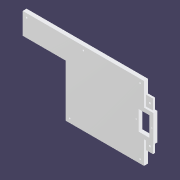
# Autodesk Inventor part: SP001b
Saved by Autodesk Inventor 2017 SP1 (Build 210196100, 196)
## iProperties
Created: 2018-01-11
Part Number: SP001b
Material: ABS Plastic
Document SubType Name: Modeling
Designer: Zach
Density: 1.06 g/cm^3
Appearance: CR White
Mass: 551.84 g
Surface Area: 1185.09 cm^2
Volume: 520.604 cm^3
Author: Zach
Autodesk Inventor part; units mm, degrees
ref_plane "YZ Plane" through (0, 0, 0) normal (1, 0, 0) x (0, 1, 0)
ref_plane "XZ Plane" through (0, 0, 0) normal (0, 1, 0) x (-1, 0, 0)
ref_plane "XY Plane" through (0, 0, 0) normal (0, 0, 1) x (1, 0, 0)
sketch "Sketch1" plane through (0, 0, 0) normal (0, 0, 1) x (1, 0, 0)
  line L0 (0, 0) -> (620, 0)
  line L1 (110, -188) -> (510, -188)
  line L2 (510, -188) -> (510, -55)
  line L3 (510, -55) -> (620, -55)
  line L4 (620, -55) -> (620, 0)
  line L5 (110, -188) -> (110, -55)
  line L6 (0, -55) -> (0, 0)
  line L7 (0, -55) -> (110, -55)
  point P0 (310, -188)
  point P1 (310, 0)
  dimension "d0" = 620
  dimension "d1" = 188
  dimension "d2" = 400
  dimension "d3" = 133
  constraints: 16 end point, 3 perpendicular, 2 horizontal, 2 midpoint, 2 parallel, 2 point on line, 1 vertical, 1 vertical alignment
  measures "d0" distance of L0.start L0.end
  measures "d1" distance between parallel lines of L0 L1
  measures "d2" distance of L1.start L1.end
  measures "d3" distance of L1.end L2.end
extrude "Extrusion1" add sketch "Sketch1" along normal blind 10
sketch "Sketch2" plane through (0, 0, 10) normal (0, 0, 1) x (1, 0, 0)
  line L0 (620, 0) -> (0, 0) projected
  line L1 (510, -188) -> (110, -188) projected
  line L2 (620, 0) -> (310, 0)
  line L3 (310, 0) -> (310, -188)
  line L4 (310, -188) -> (620, -188)
  line L5 (620, -188) -> (620, 0)
  constraints: 8 end point, 2 parallel, 1 horizontal, 1 midpoint, 1 perpendicular
extrude "Extrusion2" cut sketch "Sketch2" against normal through all
sketch "Sketch3" plane through (0, 0, 10) normal (0, 0, 1) x (1, 0, 0)
  circle A0 centre (10, -10) radius 2
  line L0 (310, 0) -> (0, 0) projected
  line L1 (0, 0) -> (0, -55) projected
  circle A1 centre (155, -10) radius 2
  circle A2 centre (300, -10) radius 2
  line L2 (310, -188) -> (310, 0) projected
  line L3 (10, -10) -> (300, -10) construction
  circle A3 centre (120, -178) radius 2
  line L4 (110, -55) -> (110, -188) projected
  line L5 (110, -188) -> (310, -188) projected
  circle A4 centre (300, -178) radius 2
  dimension "d8" = 4
  dimension "d9" = 10
  dimension "d10" = 10
  dimension "d11" = 4
  dimension "d12" = 4
  dimension "d13" = 10
  dimension "d14" = 4
  dimension "d15" = 10
  dimension "d16" = 10
  dimension "d17" = 4
  dimension "d18" = 10
  dimension "d19" = 10
  constraints: 5 centre point, 2 end point, 2 horizontal alignment, 1 coincident, 1 horizontal, 1 midpoint
  measures "d8" diameter of A0
  measures "d9" distance from line of L0 L3.start
  measures "d10" distance from line of L1 L3.start
  measures "d11" diameter of A1
  measures "d12" diameter of A2
  measures "d13" distance from line of L2 L3.end
  measures "d14" diameter of A3
  measures "d15" distance from line of L4 A3.centre
  measures "d16" distance from line of L5 A3.centre
  measures "d17" diameter of A4
  measures "d18" distance from line of L2 A4.centre
  measures "d19" distance from line of L5 A4.centre
extrude "Extrusion3" cut sketch "Sketch3" against normal through all
sketch "Sketch4" plane through (0, 0, 0) normal (0, 0, -1) x (-1, 0, 0)
  line L0 (-310, 0) -> (-310, -188) projected
  line L1 (-310, -32.5) -> (-328, -32.5)
  line L2 (-328, -32.5) -> (-328, -155.5)
  line L3 (-328, -155.5) -> (-310, -155.5)
  line L4 (-310, -155.5) -> (-310, -32.5)
  circle A0 centre (-320, -46.5) radius 2.5
  circle A1 centre (-320, -141.5) radius 2.5
  line L5 (-320, -46.5) -> (-320, -141.5) construction
  point P0 (0, 0)
  point P1 (-310, -94)
  point P2 (-320, -94)
  dimension "d22" = 18
  dimension "d23" = 123
  dimension "d24" = 5
  dimension "d25" = 5
  dimension "d26" = 10
  dimension "d27" = 95
  constraints: 10 end point, 3 midpoint, 2 centre point, 2 parallel, 1 horizontal, 1 horizontal alignment, 1 perpendicular, 1 point on line, 1 vertical, 1 vertical alignment
  measures "d22" distance of L3.end L2.end
  measures "d23" distance of L2.end L1.end
  measures "d24" diameter of A0
  measures "d25" diameter of A1
  measures "d26" distance between parallel lines of L0 L5
  measures "d27" distance of L5.start L5.end
extrude "Extrusion4" add sketch "Sketch4" against normal blind 5
sketch "Sketch6" plane through (0, 0, 10) normal (0, 0, 1) x (1, 0, 0)
  line L0 (286, -59) -> (334, -59)
  line L1 (334, -59) -> (334, -129)
  line L2 (334, -129) -> (286, -129)
  line L3 (286, -129) -> (286, -59)
  line L4 (310, -188) -> (310, 0) projected
  point P0 (0, 0)
  point P1 (310, -94)
  point P2 (310, -94)
  point P3 (286, -94)
  point P4 (310, -94)
  point P5 (310, -59)
  dimension "d42" = 48
  dimension "d43" = 70
  constraints: 8 end point, 5 midpoint, 2 parallel, 1 coincident, 1 horizontal, 1 horizontal alignment, 1 perpendicular, 1 point on line
  measures "d42" distance of L1.end L2.end
  measures "d43" distance of L0.end L1.end
extrude "Extrusion6" add sketch "Sketch6" against normal blind 10
sketch "Sketch7" plane through (0, 0, 10) normal (0, 0, 1) x (1, 0, 0)
  line L0 (324, -69) -> (296, -69)
  line L1 (296, -69) -> (296, -119)
  line L2 (296, -119) -> (324, -119)
  line L3 (324, -119) -> (324, -69)
  line L4 (310, -59) -> (310, 0) projected
  line L5 (334, -59) -> (334, -129) projected
  line L6 (290.0321, -94) -> (329.9679, -94) construction
  circle A0 centre (329.9679, -94) radius 1.5
  circle A1 centre (290.0321, -94) radius 1.5
  point P0 (0, 0)
  point P1 (324, -94)
  point P2 (334, -94)
  point P3 (310, -69)
  point P4 (310, -94)
  dimension "d46" = 28
  dimension "d47" = 50
  dimension "d50" = 39.9357
  dimension "d51" = 3
  dimension "d52" = 3
  constraints: 10 end point, 4 midpoint, 2 centre point, 2 coincident, 2 horizontal, 2 horizontal alignment, 2 parallel, 2 vertical alignment, 1 perpendicular
  measures "d46" distance of L2.end L1.end
  measures "d47" distance of L1.end L0.end
  measures "d50" distance of L6.start L6.end
  measures "d51" diameter of A0
  measures "d52" diameter of A1
extrude "Extrusion7" cut sketch "Sketch7" against normal through all
body "Solid1"
